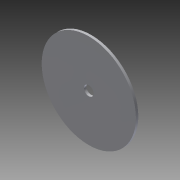
# Autodesk Inventor part: 80t Sprocket
Saved by Autodesk Inventor 2014 SP1 (Build 180222100, 222)
## iProperties
Created: 2014-02-21
Part Number: 80t Sprocket
Material: Aluminum 6061
Document SubType Name: Modeling
Designer: Asif
Density: 2.71 g/cm^3
Appearance: Aluminum - Flat
Mass: 823.599 g
Surface Area: 1011.77 cm^2
Volume: 303.911 cm^3
Author: Asif
Autodesk Inventor part; units mm, degrees
ref_plane "YZ Plane" through (0, 0, 0) normal (1, 0, 0) x (0, 1, 0)
ref_plane "XZ Plane" through (0, 0, 0) normal (0, 1, 0) x (-1, 0, 0)
ref_plane "XY Plane" through (0, 0, 0) normal (0, 0, 1) x (1, 0, 0)
sketch "Sketch1" plane through (0, 0, 0) normal (0, 0, 1) x (1, 0, 0)
  circle A0 centre (0, 0) radius 124.079
  dimension "d0" = 248.158
  constraints: 1 centre point, 1 coincident
  measures "d0" diameter of A0
extrude "Extrusion1" add sketch "Sketch1" along normal blind 6.35
sketch "Sketch2" plane through (0, 0, 6.35) normal (0, 0, 1) x (1, 0, 0)
  circle A0 centre (0, 0) radius 124.079 projected
  constraints: 1 coincident
hole "Hole1" at (0, 0, 6.35) direction (0, 0, -1) diameter 25.4 end through all
body "Solid1"
